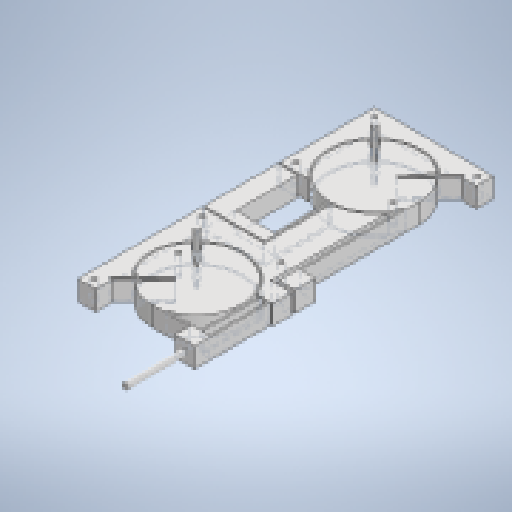
# Autodesk Inventor part: FlexK7V2
Saved by Autodesk Inventor 2023 (Build 270158000, 158)
## iProperties
Created: 2023-03-29
Part Number: FlexK7V2
Material: Generic
Document SubType Name: Modeling
Designer: Nathann
Density: 1 g/cm^3
Appearance: Default
Author: Nathann
Autodesk Inventor part; units mm, degrees
ref_plane "YZ Plane" through (0, 0, 0) normal (1, 0, 0) x (0, 1, 0)
ref_plane "XZ Plane" through (0, 0, 0) normal (0, 1, 0) x (-1, 0, 0)
ref_plane "XY Plane" through (0, 0, 0) normal (0, 0, 1) x (1, 0, 0)
sketch "Sketch1" plane through (0, 0, 0) normal (0, 1, 0) x (-1, 0, 0)
  line L0 (0, 0) -> (100, 0)
  line L1 (100, 0) -> (100, -150)
  line L2 (100, -150) -> (0, -150)
  line L3 (0, -150) -> (0, 0)
  line L4 (0, 0) -> (20, 0)
  line L5 (20, 0) -> (20, -150)
  line L6 (20, -150) -> (0, -150)
  line L7 (0, -150) -> (0, 0)
  line L8 (100, 0) -> (80, 0)
  line L9 (80, 0) -> (80, -150)
  line L10 (80, -150) -> (100, -150)
  line L11 (100, -150) -> (100, 0)
  dimension "d0" = 100
  dimension "d1" = 150
  dimension "d2" = 20
  dimension "d3" = 20
  dimension "d4" = 150
  dimension "d5" = 150
  constraints: 24 end point, 6 parallel, 3 horizontal, 3 perpendicular, 1 point on line
  measures "d0" distance of L0.start L0.end
  measures "d1" distance of L2.end L0.start
  measures "d2" distance of L9.end L10.end
  measures "d3" distance of L5.end L6.end
  measures "d4" distance of L4.end L5.end
  measures "d5" distance of L8.end L9.end
extrude "Extrusion1" add sketch "Sketch1" along normal blind 10 contours L0 L9 L2 L5
sketch "Sketch2" plane through (0, 10, 0) normal (0, 1, 0) x (1, 0, 0)
  line L0 (-80, 150) -> (-80, 0) projected
  line L1 (-80, 0) -> (-20, 0) projected
  line L2 (-20, 150) -> (-50, 120)
  line L3 (-20, 150) -> (-80, 150) projected
  line L4 (-50, 120) -> (-80, 150)
  circle A0 centre (-50, 30) radius 7.519
  circle A1 centre (-50, 120) radius 8.2469
  line L5 (-50, 120) -> (-32.764, 134.4627)
  line L6 (-50, 120) -> (-35.5373, 137.236)
  line L7 (-50, 120) -> (-64.4627, 137.236)
  line L8 (-50, 120) -> (-67.236, 134.4627)
  line L9 (-50, 30) -> (-80, 60)
  line L10 (-50, 30) -> (-64.4627, 47.236)
  line L11 (-50, 30) -> (-67.236, 44.4627)
  line L12 (-27.5, 120) -> (-27.5, 60.2126)
  line L13 (-27.5, 60.2126) -> (-20, 60.2126)
  line L14 (-80, 0) -> (-50, 30)
  line L15 (-50, 30) -> (-67.236, 15.5373)
  line L16 (-50, 30) -> (-64.4627, 12.764)
  line L17 (-49.9308, 97.5001) -> (-49.9308, 66.741)
  line L18 (-80, 66.741) -> (-80.1256, 66.741)
  line L19 (-50, 7.5) -> (-21, 7.5)
  line L20 (-21, 7.5) -> (-21, 8.5)
  line L21 (-20, 0) -> (-20, 150) projected
  line L22 (-21, 7.5) -> (-31, 7.5)
  line L23 (-31, 7.5) -> (-31, 0)
  line L24 (-31, 0) -> (-21, 0)
  line L25 (-21, 0) -> (-21, 7.5)
  line L26 (-21, 8.5) -> (-22, 8.5)
  line L27 (-22, 8.5) -> (-22, 38.5)
  line L28 (-22, 38.5) -> (-21, 38.5)
  line L29 (-21, 38.5) -> (-21, 8.5)
  line L30 (-26.5, 8.5) -> (-25.5, 8.5)
  line L31 (-25.5, 8.5) -> (-25.5, 38.5)
  line L32 (-25.5, 38.5) -> (-26.5, 38.5)
  line L33 (-26.5, 38.5) -> (-26.5, 8.5)
  line L34 (-28.5, 113.3668) -> (-28.5, 50)
  line L35 (-28.5, 50) -> (-27.5, 50)
  line L36 (-27.5, 60.2126) -> (-27.5, 120)
  line L37 (-20, 62.2126) -> (-26.5, 62.2126)
  line L38 (-27.5, 62.2126) -> (-27.5, 60.2126)
  line L39 (-27.5, 50) -> (-20, 50)
  line L40 (-20, 50) -> (-20, 62.2126)
  line L41 (-20, 50) -> (-28.5, 50)
  line L42 (-30.5318, 50) -> (-30.5318, 48)
  line L43 (-30.5318, 48) -> (-20, 48)
  line L44 (-20, 48) -> (-20, 50)
  line L45 (-28.5, 50) -> (-28.5, 106.8379)
  line L46 (-30.5318, 106.8379) -> (-30.5318, 50)
  line L47 (-26.5, 62.2126) -> (-26.5, 120)
  line L48 (-26.5, 120) -> (-27.5, 120)
  line L49 (-27.5, 120) -> (-27.5, 62.2126)
  line L50 (-49.4308, 97.5072) -> (-49.4308, 63.741)
  line L51 (-49.4308, 63.741) -> (-50.4308, 63.741)
  line L52 (-50.4308, 63.741) -> (-80, 63.741)
  line L53 (-80, 63.741) -> (-80, 69.741)
  line L54 (-80, 69.741) -> (-50.4308, 69.741)
  line L55 (-80, 69.741) -> (-70, 69.741)
  line L56 (-70, 69.741) -> (-70, 101.0864)
  line L57 (-70, 101.0864) -> (-80, 101.0864)
  line L58 (-80, 101.0864) -> (-80, 69.741)
  line L59 (-80, 63.741) -> (-49.4308, 63.741)
  line L60 (-48.4308, 63.741) -> (-48.4308, 62.741)
  line L61 (-48.4308, 62.741) -> (-80, 62.741)
  line L62 (-80, 62.741) -> (-80, 63.741)
  line L63 (-49.4308, 63.741) -> (-49.4308, 96.9392)
  line L64 (-48.4308, 96.5525) -> (-48.4308, 63.741)
  line L65 (-80, 101.0864) -> (-63.9473, 101.0864)
  line L66 (-65.2103, 102.0864) -> (-80, 102.0864)
  line L67 (-80, 102.0864) -> (-80, 101.0864)
  line L68 (-54.9514, 24.3415) -> (-71.9108, 7.382)
  line L69 (-71.9108, 7.382) -> (-72.618, 8.0892)
  line L70 (-72.618, 8.0892) -> (-55.6585, 25.0486)
  line L71 (-80, 0) -> (-71.0291, 0)
  line L72 (-71.0291, 0) -> (-71.0291, 8.9709)
  line L73 (-71.0291, 8.9709) -> (-80, 8.9709)
  line L74 (-80, 8.9709) -> (-80, 0)
  line L75 (-65.5225, 12.3562) -> (-71.0291, 6.8496)
  line L76 (-73.1504, 8.9709) -> (-67.6438, 14.4775)
  line L77 (-80, 60) -> (-71.5, 60)
  line L78 (-71.5, 60) -> (-71.5, 51.5)
  line L79 (-71.5, 51.5) -> (-80, 51.5)
  line L80 (-80, 51.5) -> (-80, 60)
  line L81 (-67.6438, 45.5225) -> (-73.6213, 51.5)
  line L82 (-65.5225, 47.6438) -> (-71.5, 53.6213)
  line L83 (-54.9514, 35.6585) -> (-71.5, 52.2071)
  line L84 (-72.2071, 51.5) -> (-55.6585, 34.9514)
  line L85 (-56.1742, 125.4671) -> (-72.2071, 141.5)
  line L86 (-80, 150) -> (-71.5, 150)
  line L87 (-71.5, 150) -> (-71.5, 141.5)
  line L88 (-71.5, 141.5) -> (-80, 141.5)
  line L89 (-80, 141.5) -> (-80, 150)
  line L90 (-20, 150) -> (-28.5, 150)
  line L91 (-28.5, 150) -> (-28.5, 141.5)
  line L92 (-28.5, 141.5) -> (-20, 141.5)
  line L93 (-20, 141.5) -> (-20, 150)
  line L94 (-55.4671, 126.1742) -> (-71.5, 142.2071)
  line L95 (-73.6213, 141.5) -> (-67.6438, 135.5225)
  line L96 (-65.5225, 137.6438) -> (-71.5, 143.6213)
  line L97 (-43.8258, 125.4671) -> (-27.7929, 141.5)
  line L98 (-44.5329, 126.1742) -> (-28.5, 142.2071)
  line L99 (-32.3562, 135.5225) -> (-26.3787, 141.5)
  line L100 (-34.4775, 137.6438) -> (-28.5, 143.6213)
  line L101 (-21, 8.5) -> (-25.5, 8.5)
  line L102 (-26.5, 8.5) -> (-43.3668, 8.5)
  line L103 (-22, 38.5) -> (-25.5, 38.5)
  line L104 (-26.5, 38.5) -> (-28.0911, 38.5)
  line L105 (-21, 38.5) -> (-20, 38.5)
  line L106 (-20, 38.5) -> (-20, 0)
  line L107 (-20, 0) -> (-21, 0)
  line L108 (-21, 0) -> (-21, 38.5)
  line L109 (-80, 0) -> (-20, 0)
  line L110 (-20, 0) -> (-20, 150)
  line L111 (-20, 150) -> (-80, 150)
  line L112 (-80, 150) -> (-80, 0)
  arc A2 (-65.5225, 12.3562) -> (-43.2177, 7.5) centre (-50, 30) ccw
  arc A3 (-66.9668, 13.7403) -> (-66.2597, 13.0332) centre (-50, 30) ccw
  arc A4 (-64.4627, 12.764) -> (-50, 7.5) centre (-50, 30) ccw
  arc A5 (-66.2595, 14.4476) -> (-65.5524, 13.7405) centre (-50, 30) ccw
  arc A6 (-67.236, 44.4627) -> (-67.236, 15.5373) centre (-50, 30) ccw
  arc A7 (-43.3668, 8.5) -> (-64.4627, 47.236) centre (-50, 30) ccw
  arc A8 (-65.5524, 46.2595) -> (-66.2595, 45.5524) centre (-50, 30) ccw
  arc A9 (-40.5132, 8.5) -> (-65.5225, 47.6438) centre (-50, 30) ccw
  arc A10 (-66.2597, 46.9668) -> (-66.9668, 46.2597) centre (-50, 30) ccw
  arc A11 (-67.6438, 45.5225) -> (-67.6438, 14.4775) centre (-50, 30) ccw
  arc A12 (-27.5, 120) -> (-32.764, 134.4627) centre (-50, 120) ccw
  arc A13 (-33.7405, 135.5524) -> (-34.4476, 136.2595) centre (-50, 120) ccw
  arc A14 (-26.5, 120) -> (-32.3562, 135.5225) centre (-50, 120) ccw
  arc A15 (-33.0332, 136.2597) -> (-33.7403, 136.9668) centre (-50, 120) ccw
  arc A16 (-35.5373, 137.236) -> (-64.4627, 137.236) centre (-50, 120) ccw
  arc A17 (-65.5524, 136.2595) -> (-66.2595, 135.5524) centre (-50, 120) ccw
  arc A18 (-34.4775, 137.6438) -> (-65.5225, 137.6438) centre (-50, 120) ccw
  arc A19 (-66.2597, 136.9668) -> (-66.9668, 136.2597) centre (-50, 120) ccw
  arc A20 (-67.6438, 135.5225) -> (-65.2103, 102.0864) centre (-50, 120) ccw
  line L113 (-50.4308, 69.741) -> (-50.4308, 97.5041)
  arc A21 (-48.4308, 96.5525) -> (-30.5318, 106.8379) centre (-50, 120) ccw
  arc A22 (-63.9473, 101.0864) -> (-50.4308, 96.5039) centre (-50, 120) ccw
  arc A23 (-67.236, 134.4627) -> (-50.4308, 97.5041) centre (-50, 120) ccw
  arc A24 (-49.4308, 97.5072) -> (-28.5, 113.3668) centre (-50, 120) ccw
  point P0 (-56.3175, 125.301)
  point P1 (-44.699, 126.3175)
  point P2 (-55.301, 126.3175)
  point P3 (-43.6825, 125.301)
  point P4 (-54.8331, 24.2401)
  point P5 (-71.0291, 8.2638)
  point P6 (-55.7599, 34.8331)
  point P7 (-71.7362, 8.9709)
  point P8 (-55.7599, 25.1669)
  point P9 (-54.8331, 35.7599)
  dimension "d23" = 1
  dimension "d25" = 10
  dimension "d26" = 30
  dimension "d27" = 1
  dimension "d28" = 1
  dimension "d29" = 1
  dimension "d31" = 50
  dimension "d32" = 7.5
  dimension "d34" = 2
  dimension "d35" = 2
  dimension "d37" = 0.5
  dimension "d39" = 3
  dimension "d40" = 3
  dimension "d41" = 45
  dimension "d43" = 30
  dimension "d44" = 45
  dimension "d45" = 10
  dimension "d46" = 1
  dimension "d47" = 1
  dimension "d48" = 1
  dimension "d49" = 0.5
  dimension "d50" = 0.5
  dimension "d51" = 1
  dimension "d52" = 1
  dimension "d53" = 8.5
  dimension "d58" = 0.5
  dimension "d59" = 0.5
  dimension "d60" = 1
  dimension "d61" = 1
  dimension "d62" = 0.5
  dimension "d63" = 0.5
  dimension "d64" = 1
  dimension "d65" = 1
  dimension "d66" = 8.5
  dimension "d67" = 8.5
  dimension "d68" = 30
  dimension "d69" = 30
  dimension "d70" = 30
  dimension "d71" = 8.5
  dimension "d72" = 8.5
  dimension "d73" = 0.5
  dimension "d74" = 0.5
  dimension "d75" = 1
  dimension "d76" = 1
  dimension "d77" = 5
  dimension "d78" = 5
  dimension "d79" = 5
  dimension "d80" = 5
  dimension "d81" = 5
  dimension "d82" = 5
  dimension "d83" = 5
  dimension "d84" = 5
  constraints: 220 end point, 55 point on circle, 49 parallel, 46 point on line, 25 centre point, 20 perpendicular, 16 horizontal, 4 coincident, 2 vertical, 1 collinear
  measures "d23" distance between parallel lines of L20 L21
  measures "d25" distance of L23.end L24.end
  measures "d26" distance of L26.end L27.end
  measures "d27" distance between parallel lines of L31 L33
  measures "d28" distance between parallel lines of L27 L29
  measures "d29" distance between parallel lines of L34 L36
  measures "d31" distance between parallel lines of L1 L39
  measures "d32" distance between parallel lines of L38 L40
  measures "d34" distance between parallel lines of L39 L43
  measures "d35" distance between parallel lines of L37 L13
  measures "d37" distance between parallel lines of L17 L50
  measures "d39" distance between parallel lines of L18 L52
  measures "d40" distance between parallel lines of L54 L18
  measures "d41" angle of L0 L14
  measures "d43" distance from line of L21 A4.centre
  measures "d44" angle of L0 L9
  measures "d45" distance between parallel lines of L0 L56
  measures "d46" distance between parallel lines of L61 L52
  measures "d47" distance between parallel lines of L64 L63
  measures "d48" distance between parallel lines of L66 L65
  measures "d49" distance between parallel lines of L68 L14
  measures "d50" distance between parallel lines of L70 L14
  measures "d51" distance between parallel lines of L75 L68
  measures "d52" distance between parallel lines of L76 L70
  measures "d53" distance of L77.end L78.end
  measures "d58" distance between parallel lines of L9 L84
  measures "d59" distance between parallel lines of L9 L83
  measures "d60" distance between parallel lines of L84 L81
  measures "d61" distance between parallel lines of L83 L82
  measures "d62" distance between parallel lines of L85 L4
  measures "d63" distance between parallel lines of L4 L94
  measures "d64" distance between parallel lines of L95 L85
  measures "d65" distance between parallel lines of L96 L94
  measures "d66" distance of L86.end L87.end
  measures "d67" distance of L87.end L88.end
  measures "d68" distance from line of L21 A12.centre
  measures "d69" distance from line of L3 A12.centre
  measures "d70" distance from line of L1 A4.centre
  measures "d71" distance of L90.end L91.end
  measures "d72" distance of L91.end L92.end
  measures "d73" distance between parallel lines of L2 L97
  measures "d74" distance between parallel lines of L98 L2
  measures "d75" distance between parallel lines of L100 L98
  measures "d76" distance between parallel lines of L99 L97
  measures "d77" angle of L15 L70
  measures "d78" angle of L16 L68
  measures "d79" angle of L11 L84
  measures "d80" angle of L10 L83
  measures "d81" angle of L8 L85
  measures "d82" angle of L7 L94
  measures "d83" angle of L6 L98
  measures "d84" angle of L97 L5
extrude "Extrusion2" cut sketch "Sketch2" against normal blind 20 contours L66 A20 L95 L88 L85 A1 L8 A23 L113 A22 L65 L57 L0 | L96 A18 L100 L91 L98 A1 L6 A16 L7 L94 L87 | L65 A22 L113 L54 L56 | L21 L37 L47 A14 L99 L92 | L92 L99 A14 L48 A12 L5 A1 L97 | L21 L13 L12 L48 L47 L37 | L52 L51 L50 A24 L34 L35 L39 L21 L43 L42 L46 A21 L64 L60 L61 L0 | L21 L1 L25 L20 L29 L105 | L79 L84 A0 L11 A6 L15 L70 L73 L76 A11 L81 | L78 L82 A9 L102 A7 L10 A0 L83 | L27 L101 L31 L103 | L72 L75 A2 L19 L23 L1 | L104 L33 A9 | L72 L68 A0 L16 A4 L19 A2 L75 | L33 L102 A9
sketch "Sketch6" plane through (0, 10, 0) normal (0, 1, 0) x (1, 0, 0)
  arc A0 (-43.3668, 8.5) -> (-64.4627, 47.236) centre (-50, 30) ccw projected
  arc A1 (-49.4308, 97.5072) -> (-28.5, 113.3668) centre (-50, 120) ccw projected
  arc A2 (-43.3668, 8.5) -> (-64.4627, 47.236) centre (-50, 30) ccw projected
  arc A3 (-49.4308, 97.5072) -> (-28.5, 113.3668) centre (-50, 120) ccw projected
  line L0 (-28.5, 113.3668) -> (-28.5, 50) projected
  line L1 (-48.4308, 62.741) -> (-80, 62.741) projected
  line L2 (-30.5318, 106.8379) -> (-30.5318, 48) projected
  arc A4 (-67.236, 44.4627) -> (-67.236, 15.5373) centre (-50, 30) ccw projected
  line L3 (-72.5, 30) -> (-27.5, 120)
  circle A5 centre (-76, 4) radius 1.325
  circle A6 centre (-76, 58.741) radius 1.325
  circle A7 centre (-36, 58.741) radius 1.325
  circle A8 centre (-24, 146) radius 1.325
  circle A9 centre (-76, 146) radius 1.325
  circle A10 centre (-76, 106.0864) radius 1.325
  line L4 (-80, 0) -> (-71.0291, 0) projected
  line L5 (-80, 62.741) -> (-80, 0) projected
  line L6 (-20, 141.5) -> (-20, 150) projected
  line L7 (-20, 150) -> (-80, 150) projected
  line L8 (-80, 150) -> (-80, 102.0864) projected
  line L9 (-80, 102.0864) -> (-65.2103, 102.0864) projected
  point P0 (0, 0)
  dimension "d94" = 4
  dimension "d95" = 4
  dimension "d96" = 2.65
  dimension "d97" = 4
  dimension "d98" = 4
  dimension "d99" = 2.65
  dimension "d100" = 0
  dimension "d101" = 2.65
  dimension "d102" = 40
  dimension "d103" = 2.65
  dimension "d104" = 2.65
  dimension "d105" = 2.65
  dimension "d106" = 4
  dimension "d107" = 4
  dimension "d108" = 4
  dimension "d109" = 4
  dimension "d110" = 4
  dimension "d111" = 4
  constraints: 6 centre point, 2 end point, 1 point on circle
  measures "d94" distance from line of L4 A5.centre
  measures "d95" distance from line of A5.centre L5
  measures "d96" diameter of A5
  measures "d97" distance from line of L5 A6.centre
  measures "d98" distance from line of L1 A6.centre
  measures "d99" diameter of A6
  measures "d100" vertical distance of A7.centre A6.centre
  measures "d101" diameter of A7
  measures "d102" distance of A6.centre A7.centre
  measures "d103" diameter of A10
  measures "d104" diameter of A9
  measures "d105" diameter of A8
  measures "d106" distance from line of L6 A8.centre
  measures "d107" distance from line of L7 A8.centre
  measures "d108" distance from line of L7 A9.centre
  measures "d109" distance from line of L8 A9.centre
  measures "d110" distance from line of L9 A10.centre
  measures "d111" distance from line of L8 A10.centre
extrude "Extrusion3" cut sketch "Sketch6" against normal blind 10
sketch "Sketch7" plane through (0, 10, 0) normal (0, 1, 0) x (1, 0, 0)
  circle A0 centre (-66.1225, 36.8056) radius 1.1 projected
  circle A1 centre (-33.8775, 113.1944) radius 1.1 projected
  circle A2 centre (-66.1225, 36.8056) radius 1.325
  circle A3 centre (-33.8775, 113.1944) radius 1.325
  point P0 (0, 0)
  dimension "d114" = 2.65
  dimension "d115" = 2.65
  constraints: 2 centre point, 2 coincident
  measures "d114" diameter of A3
  measures "d115" diameter of A2
extrude "Extrusion4" cut sketch "Sketch7" against normal blind 10 contours A0 | A1 | A2 | A3
sketch "Sketch8" plane through (-31, 0, 0) normal (0, 0, 1) x (1, 0, 0)
  circle A0 centre (5, 5) radius 1.5
  line L0 (0, 10) -> (10, 10) projected
  line L1 (10, 0) -> (10, 10) projected
  point P0 (31, 0)
  dimension "d118" = 3
  dimension "d119" = 5
  dimension "d120" = 5
  constraints: 1 centre point
  measures "d118" diameter of A0
  measures "d119" distance from line of L0 A0.centre
  measures "d120" distance from line of L1 A0.centre
extrude "Extrusion5" add sketch "Sketch8" along normal blind 30
equation "\"d27\" = d24"
equation "\"d28\" = BladeThickness"
equation "\"d29\" = d27"
equation "\"d37\" = d36"
equation "\"d49\" = 0.5 * d24"
equation "\"d50\" = d49"
equation "\"d58\" = 0.5 * d24"
equation "\"d59\" = d58"
equation "\"d61\" = d60"
equation "\"d62\" = 0.5 * d24"
equation "\"d63\" = d62"
equation "\"d73\" = d63"
equation "\"d74\" = d73"
equation "\"d19\" = d18"
equation "\"d21\" = d22"
equation "\"d24\" = BladeThickness"
equation "\"BladeThickness\" = 1"
equation "\"NeckThickness\" = 1"
equation "\"d36\" = 0.5 * d27"
equation "\"d18\" = 45"
equation "\"d22\" = 47"
body "Solid1"
